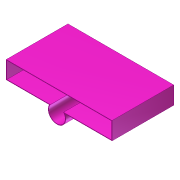
# Autodesk Inventor part: LauncherMockup
Saved by Autodesk Inventor 2012 (Build 160160000, 160)
## iProperties
Created: 2013-01-12
Part Number: LauncherMockup
Material: Default
Document SubType Name: Modeling
Designer: JesseK
Density: 1 g/cm^3
Author: JesseK
Autodesk Inventor part; units mm, degrees
ref_plane "YZ Plane" through (0, 0, 0) normal (1, 0, 0) x (0, 1, 0)
ref_plane "XZ Plane" through (0, 0, 0) normal (0, 1, 0) x (-1, 0, 0)
ref_plane "XY Plane" through (0, 0, 0) normal (0, 0, 1) x (1, 0, 0)
sketch "Sketch1" plane through (0, 0, 0) normal (0, 0, 1) x (1, 0, 0)
  line L0 (584.2, 0) -> (584.2, 101.6)
  line L1 (584.2, 101.6) -> (0, 101.6)
  line L2 (0, 101.6) -> (0, 0)
  line L3 (0, 0) -> (159.2059, 0)
  line L4 (247.1941, 0) -> (584.2, 0)
  arc A0 (159.2059, 0) -> (247.1941, 0) centre (203.2, -25.4) ccw
  dimension "d2" = 101.6
  dimension "d4" = 203.2
  dimension "d5" = 50.8
  dimension "d6" = 25.4
  dimension "d8" = 584.2
  constraints: 11 end point, 2 horizontal, 2 point on circle, 1 centre point, 1 collinear, 1 parallel, 1 perpendicular
  measures "d2" distance of L1.end L2.end
  measures "d4" horizontal distance of A0.centre L2.end
  measures "d5" radius of A0
  measures "d6" vertical distance of L2.end A0.centre
  measures "d8" distance of L0.end L1.end
extrude "Extrusion1" add sketch "Sketch1" along normal blind 355.6
shell "Shell1" thickness 3.175 removed faces 2 at (277.1314, 67.7333, 0) at (277.1314, 67.7333, 355.6)
body "Solid1"
